Autodesk Fusion 360 part; units mm, degrees
(part 2 of 5)
  spline S371 degree 3 poles (-22.5351, -2.4516) (-22.49, -2.4245) (-22.4449, -2.4426) (-22.4449, -2.4877) knots 0 0 0 0 1 1 1 1
  spline S372 degree 3 poles (-22.4449, -2.4877) (-22.4449, -2.5419) (-22.49, -2.587) (-22.5351, -2.587) knots 0 0 0 0 1 1 1 1
  spline S373 degree 3 poles (-22.5351, -2.587) (-22.5893, -2.587) (-22.6254, -2.5689) (-22.6254, -2.5509) knots 0 0 0 0 1 1 1 1
  spline S374 degree 3 poles (-18.0948, -1.7747) (-17.9685, -1.7386) (-17.806, -1.6755) (-17.7338, -1.6303) knots 0 0 0 0 1 1 1 1
  spline S375 degree 3 poles (-17.7338, -1.6303) (-17.6436, -1.5762) (-17.6436, -1.5942) (-17.7429, -1.7116) knots 0 0 0 0 1 1 1 1
  spline S376 degree 3 poles (-17.7429, -1.7116) (-17.806, -1.7928) (-17.9685, -1.865) (-18.1039, -1.856) knots 0 0 0 0 1 1 1 1
  line L50 (-18.1039, -1.856) -> (-18.3385, -1.8469)
  line L51 (-18.3385, -1.8469) -> (-18.0948, -1.7747)
  spline S377 degree 3 poles (-20.1345, -1.7838) (-20.1616, -1.7386) (-20.0533, -1.6845) (-19.8908, -1.6574) knots 0 0 0 0 1 1 1 1
  spline S378 degree 3 poles (-19.8908, -1.6574) (-19.5569, -1.6123) (-19.4576, -1.6574) (-19.6471, -1.7747) knots 0 0 0 0 1 1 1 1
  spline S379 degree 3 poles (-19.6471, -1.7747) (-19.8186, -1.883) (-20.0713, -1.8921) (-20.1345, -1.7838) knots 0 0 0 0 1 1 1 1
  spline S380 degree 3 poles (-21.9034, -1.6845) (-22.0027, -1.6213) (-21.9666, -1.5942) (-21.7409, -1.5942) knots 0 0 0 0 1 1 1 1
  spline S381 degree 3 poles (-21.7409, -1.5942) (-21.5604, -1.5942) (-21.4612, -1.6303) (-21.4973, -1.6845) knots 0 0 0 0 1 1 1 1
  spline S382 degree 3 poles (-21.4973, -1.6845) (-21.5695, -1.8018) (-21.7319, -1.8018) (-21.9034, -1.6845) knots 0 0 0 0 1 1 1 1
  spline S383 degree 3 poles (-27.887, -1.5401) (-28.7714, -1.3957) (-29.1595, -1.2332) (-29.3129, -0.9444) knots 0 0 0 0 1 1 1 1
  spline S384 degree 3 poles (-29.3129, -0.9444) (-29.4032, -0.782) (-29.3851, -0.7278) (-29.2497, -0.6286) knots 0 0 0 0 1 1 1 1
  spline S385 degree 3 poles (-29.2497, -0.6286) (-29.1053, -0.5203) (-29.0692, -0.5383) (-28.97, -0.7369) knots 0 0 0 0 1 1 1 1
  spline S386 degree 3 poles (-28.97, -0.7369) (-28.8887, -0.8813) (-28.7714, -0.9625) (-28.636, -0.9625) knots 0 0 0 0 1 1 1 1
  spline S387 degree 3 poles (-28.636, -0.9625) (-28.5187, -0.9625) (-28.3021, -1.0257) (-28.1667, -1.0979) knots 0 0 0 0 1 1 1 1
  spline S388 degree 3 poles (-28.1667, -1.0979) (-27.8689, -1.2513) (-26.9935, -1.2784) (-26.9123, -1.143) knots 0 0 0 0 1 1 1 1
  spline S389 degree 3 poles (-26.9123, -1.143) (-26.8762, -1.0888) (-27.0386, -1.0527) (-27.3455, -1.0527) knots 0 0 0 0 1 1 1 1
  spline S390 degree 3 poles (-27.3455, -1.0527) (-27.7065, -1.0527) (-27.8689, -1.0076) (-27.9862, -0.8813) knots 0 0 0 0 1 1 1 1
  spline S391 degree 3 poles (-27.9862, -0.8813) (-28.0765, -0.791) (-28.2841, -0.6827) (-28.4555, -0.6556) knots 0 0 0 0 1 1 1 1
  spline S392 degree 3 poles (-28.4555, -0.6556) (-28.8346, -0.5834) (-28.8436, -0.4481) (-28.4916, -0.06) knots 0 0 0 0 1 1 1 1
  spline S393 degree 3 poles (-28.4916, -0.06) (-28.3382, 0.1115) (-28.1938, 0.3461) (-28.1577, 0.4635) knots 0 0 0 0 1 1 1 1
  spline S394 degree 3 poles (-28.1577, 0.4635) (-28.1126, 0.644) (-28.0675, 0.662) (-27.8689, 0.6079) knots 0 0 0 0 1 1 1 1
  spline S395 degree 3 poles (-27.8689, 0.6079) (-27.7426, 0.5718) (-27.526, 0.5537) (-27.3816, 0.5627) knots 0 0 0 0 1 1 1 1
  spline S396 degree 3 poles (-27.3816, 0.5627) (-27.0928, 0.5808) (-26.7137, 0.3552) (-26.6686, 0.1386) knots 0 0 0 0 1 1 1 1
  spline S397 degree 3 poles (-26.6686, 0.1386) (-26.6325, -0.069) (-25.748, -0.0961) (-24.8907, 0.0934) knots 0 0 0 0 1 1 1 1
  spline S398 degree 3 poles (-24.8907, 0.0934) (-24.2679, 0.2288) (-24.2048, 0.2288) (-23.9611, 0.0754) knots 0 0 0 0 1 1 1 1
  spline S399 degree 3 poles (-23.9611, 0.0754) (-23.7535, -0.0419) (-23.6633, -0.051) (-23.5911, 0.0303) knots 0 0 0 0 1 1 1 1
  spline S400 degree 3 poles (-23.5911, 0.0303) (-23.5098, 0.1115) (-23.5189, 0.1566) (-23.6452, 0.2469) knots 0 0 0 0 1 1 1 1
  spline S401 degree 3 poles (-23.6452, 0.2469) (-23.8347, 0.3913) (-23.8347, 0.4454) (-23.6633, 0.5176) knots 0 0 0 0 1 1 1 1
  spline S402 degree 3 poles (-23.6633, 0.5176) (-23.5279, 0.5627) (-23.0766, 0.1927) (-23.0766, 0.0303) knots 0 0 0 0 1 1 1 1
  spline S403 degree 3 poles (-23.0766, 0.0303) (-23.0766, -0.078) (-22.9774, -0.078) (-22.8149, 0.0212) knots 0 0 0 0 1 1 1 1
  spline S404 degree 3 poles (-22.8149, 0.0212) (-22.7517, 0.0664) (-22.7247, 0.1476) (-22.7517, 0.2017) knots 0 0 0 0 1 1 1 1
  spline S405 degree 3 poles (-22.7517, 0.2017) (-22.7878, 0.2559) (-22.7247, 0.3371) (-22.5893, 0.3913) knots 0 0 0 0 1 1 1 1
  spline S406 degree 3 poles (-22.5893, 0.3913) (-22.3185, 0.4905) (-22.2915, 0.7071) (-22.499, 0.9418) knots 0 0 0 0 1 1 1 1
  spline S407 degree 3 poles (-22.499, 0.9418) (-22.6344, 1.0862) (-22.6254, 1.1313) (-22.3456, 1.4652) knots 0 0 0 0 1 1 1 1
  spline S408 degree 3 poles (-22.3456, 1.4652) (-22.1832, 1.6728) (-21.9846, 1.8353) (-21.9034, 1.8353) knots 0 0 0 0 1 1 1 1
  spline S409 degree 3 poles (-21.9034, 1.8353) (-21.6687, 1.8353) (-21.4973, 2.0789) (-21.6236, 2.2324) knots 0 0 0 0 1 1 1 1
  spline S410 degree 3 poles (-21.6236, 2.2324) (-21.8131, 2.458) (-21.4251, 3.8027) (-21.1543, 3.8388) knots 0 0 0 0 1 1 1 1
  spline S411 degree 3 poles (-21.1543, 3.8388) (-21.1002, 3.8388) (-19.9901, 3.8569) (-18.6995, 3.8659) knots 0 0 0 0 1 1 1 1
  spline S412 degree 3 poles (-18.6995, 3.8659) (-17.4089, 3.8749) (-15.8566, 3.92) (-15.261, 3.9561) knots 0 0 0 0 1 1 1 1
  spline S413 degree 3 poles (-15.261, 3.9561) (-14.6563, 3.9922) (-14.0877, 4.0013) (-14.0065, 3.9652) knots 0 0 0 0 1 1 1 1
  spline S414 degree 3 poles (-14.0065, 3.9652) (-13.8531, 3.911) (-13.8531, 3.902) (-13.9975, 3.7395) knots 0 0 0 0 1 1 1 1
  spline S415 degree 3 poles (-13.9975, 3.7395) (-14.187, 3.532) (-14.3134, 3.4959) (-15.5678, 3.3334) knots 0 0 0 0 1 1 1 1
  spline S416 degree 3 poles (-15.5678, 3.3334) (-16.5967, 3.198) (-17.1111, 3.0085) (-17.436, 2.6475) knots 0 0 0 0 1 1 1 1
  spline S417 degree 3 poles (-17.436, 2.6475) (-17.7158, 2.3316) (-19.3222, 1.5645) (-19.6923, 1.5645) knots 0 0 0 0 1 1 1 1
  spline S418 degree 3 poles (-19.6923, 1.5645) (-20.0172, 1.5645) (-20.5496, 1.3479) (-20.5496, 1.2216) knots 0 0 0 0 1 1 1 1
  spline S419 degree 3 poles (-20.5496, 1.2216) (-20.5496, 1.1855) (-20.6399, 1.1133) (-20.7572, 1.0681) knots 0 0 0 0 1 1 1 1
  spline S420 degree 3 poles (-20.7572, 1.0681) (-20.8655, 1.014) (-21.0641, 0.7613) (-21.1994, 0.4905) knots 0 0 0 0 1 1 1 1
  spline S421 degree 3 poles (-21.1994, 0.4905) (-21.5334, -0.1683) (-21.8131, -0.439) (-22.5351, -0.8181) knots 0 0 0 0 1 1 1 1
  spline S422 degree 3 poles (-22.5351, -0.8181) (-23.1398, -1.143) (-24.4665, -1.6394) (-24.8816, -1.7025) knots 0 0 0 0 1 1 1 1
  spline S423 degree 3 poles (-24.8816, -1.7025) (-25.2878, -1.7747) (-27.0747, -1.6755) (-27.887, -1.5401) knots 0 0 0 0 1 1 1 1
  spline S424 degree 3 poles (-18.0226, -1.4589) (-17.9595, -1.3867) (-17.8692, -1.3235) (-17.8241, -1.3235) knots 0 0 0 0 1 1 1 1
  spline S425 degree 3 poles (-17.8241, -1.3235) (-17.7699, -1.3235) (-17.779, -1.3867) (-17.8421, -1.4589) knots 0 0 0 0 1 1 1 1
  spline S426 degree 3 poles (-17.8421, -1.4589) (-17.9053, -1.5311) (-17.9956, -1.5942) (-18.0407, -1.5942) knots 0 0 0 0 1 1 1 1
  spline S427 degree 3 poles (-18.0407, -1.5942) (-18.0948, -1.5942) (-18.0858, -1.5311) (-18.0226, -1.4589) knots 0 0 0 0 1 1 1 1
  spline S428 degree 3 poles (-20.0081, -1.5581) (-20.0081, -1.5401) (-19.945, -1.495) (-19.8637, -1.4679) knots 0 0 0 0 1 1 1 1
  spline S429 degree 3 poles (-19.8637, -1.4679) (-19.7915, -1.4408) (-19.7554, -1.4498) (-19.7825, -1.504) knots 0 0 0 0 1 1 1 1
  spline S430 degree 3 poles (-19.7825, -1.504) (-19.8367, -1.5942) (-20.0081, -1.6303) (-20.0081, -1.5581) knots 0 0 0 0 1 1 1 1
  spline S431 degree 3 poles (-18.3836, -1.3506) (-18.3114, -1.3235) (-18.167, -1.2603) (-18.0678, -1.2062) knots 0 0 0 0 1 1 1 1
  spline S432 degree 3 poles (-18.0678, -1.2062) (-17.9053, -1.1249) (-17.8963, -1.1249) (-18.0136, -1.2603) knots 0 0 0 0 1 1 1 1
  spline S433 degree 3 poles (-18.0136, -1.2603) (-18.0768, -1.3506) (-18.2212, -1.4137) (-18.3295, -1.4047) knots 0 0 0 0 1 1 1 1
  spline S434 degree 3 poles (-18.3295, -1.4047) (-18.4558, -1.4047) (-18.4739, -1.3867) (-18.3836, -1.3506) knots 0 0 0 0 1 1 1 1
  spline S435 degree 3 poles (-20.324, -1.3325) (-20.2699, -1.2964) (-20.1164, -1.2332) (-19.963, -1.1971) knots 0 0 0 0 1 1 1 1
  spline S436 degree 3 poles (-19.963, -1.1971) (-19.7103, -1.143) (-19.7013, -1.152) (-19.8637, -1.2784) knots 0 0 0 0 1 1 1 1
  spline S437 degree 3 poles (-19.8637, -1.2784) (-20.0533, -1.4228) (-20.4684, -1.4769) (-20.324, -1.3325) knots 0 0 0 0 1 1 1 1
  spline S438 degree 3 poles (-21.8402, -1.3506) (-21.777, -1.3325) (-21.6687, -1.3325) (-21.6146, -1.3506) knots 0 0 0 0 1 1 1 1
  spline S439 degree 3 poles (-21.6146, -1.3506) (-21.5514, -1.3776) (-21.5965, -1.3957) (-21.7229, -1.3957) knots 0 0 0 0 1 1 1 1
  spline S440 degree 3 poles (-21.7229, -1.3957) (-21.8492, -1.3957) (-21.8944, -1.3776) (-21.8402, -1.3506) knots 0 0 0 0 1 1 1 1
  spline S441 degree 3 poles (17.4817, -1.0979) (16.2363, -0.8452) (15.8662, -0.6286) (15.3518, 0.1205) knots 0 0 0 0 1 1 1 1
  spline S442 degree 3 poles (15.3518, 0.1205) (14.9096, 0.7703) (14.5125, 1.6096) (14.4313, 2.0609) knots 0 0 0 0 1 1 1 1
  spline S443 degree 3 poles (14.4313, 2.0609) (14.3952, 2.2594) (14.2688, 2.5663) (14.1515, 2.7378) knots 0 0 0 0 1 1 1 1
  spline S444 degree 3 poles (14.1515, 2.7378) (13.9981, 2.9724) (13.9259, 3.2432) (13.8807, 3.7486) knots 0 0 0 0 1 1 1 1
  line L52 (13.8807, 3.7486) -> (13.8176, 4.4525)
  line L53 (13.8176, 4.4525) -> (14.0973, 4.4525)
  spline S445 degree 3 poles (14.0973, 4.4525) (14.6749, 4.4525) (14.7381, 4.3532) (14.7381, 3.4778) knots 0 0 0 0 1 1 1 1
  spline S446 degree 3 poles (14.7381, 3.4778) (14.7381, 3.0266) (14.693, 2.6385) (14.6388, 2.5843) knots 0 0 0 0 1 1 1 1
  spline S447 degree 3 poles (14.6388, 2.5843) (14.5305, 2.476) (14.8013, 1.8533) (15.0991, 1.5194) knots 0 0 0 0 1 1 1 1
  spline S448 degree 3 poles (15.0991, 1.5194) (15.1803, 1.4201) (15.3338, 1.2216) (15.424, 1.0681) knots 0 0 0 0 1 1 1 1
  spline S449 degree 3 poles (15.424, 1.0681) (15.5774, 0.8245) (15.5865, 0.8064) (15.433, 0.8696) knots 0 0 0 0 1 1 1 1
  spline S450 degree 3 poles (15.433, 0.8696) (15.3247, 0.9057) (15.2796, 0.8876) (15.2796, 0.7884) knots 0 0 0 0 1 1 1 1
  spline S451 degree 3 poles (15.2796, 0.7884) (15.2796, 0.6801) (15.3338, 0.653) (15.4872, 0.6891) knots 0 0 0 0 1 1 1 1
  spline S452 degree 3 poles (15.4872, 0.6891) (15.5955, 0.7252) (15.7489, 0.7071) (15.8211, 0.662) knots 0 0 0 0 1 1 1 1
  spline S453 degree 3 poles (15.8211, 0.662) (15.9114, 0.5988) (15.9204, 0.5718) (15.8392, 0.5718) knots 0 0 0 0 1 1 1 1
  spline S454 degree 3 poles (15.8392, 0.5718) (15.6587, 0.5718) (15.7218, 0.4454) (15.9655, 0.3281) knots 0 0 0 0 1 1 1 1
  spline S455 degree 3 poles (15.9655, 0.3281) (16.0919, 0.2739) (16.2543, 0.2469) (16.3265, 0.2739) knots 0 0 0 0 1 1 1 1
  spline S456 degree 3 poles (16.3265, 0.2739) (16.3987, 0.301) (16.507, 0.283) (16.5702, 0.2288) knots 0 0 0 0 1 1 1 1
  spline S457 degree 3 poles (16.5702, 0.2288) (16.6243, 0.1837) (17.0034, 0.0122) (17.4005, -0.1502) knots 0 0 0 0 1 1 1 1
  spline S458 degree 3 poles (17.4005, -0.1502) (18.0593, -0.412) (18.1947, -0.43) (19.0701, -0.421) knots 0 0 0 0 1 1 1 1
  spline S459 degree 3 poles (19.0701, -0.421) (19.5936, -0.412) (20.126, -0.412) (20.2614, -0.421) knots 0 0 0 0 1 1 1 1
  spline S460 degree 3 poles (20.2614, -0.421) (20.6765, -0.439) (21.1097, -0.3939) (20.9744, -0.3488) knots 0 0 0 0 1 1 1 1
  spline S461 degree 3 poles (20.9744, -0.3488) (20.8841, -0.3217) (20.9022, -0.2585) (21.0646, -0.1322) knots 0 0 0 0 1 1 1 1
  spline S462 degree 3 poles (21.0646, -0.1322) (21.218, -0.0058) (21.2361, 0.0303) (21.1188, -0.0058) knots 0 0 0 0 1 1 1 1
  spline S463 degree 3 poles (21.1188, -0.0058) (20.83, -0.0961) (20.848, 0.1927) (21.1458, 0.5627) knots 0 0 0 0 1 1 1 1
  spline S464 degree 3 poles (21.1458, 0.5627) (21.3805, 0.8425) (21.5068, 0.9328) (21.7686, 0.9508) knots 0 0 0 0 1 1 1 1
  spline S465 degree 3 poles (21.7686, 0.9508) (22.0574, 0.9779) (22.0935, 1.005) (22.0754, 1.2216) knots 0 0 0 0 1 1 1 1
  spline S466 degree 3 poles (22.0754, 1.2216) (22.0664, 1.393) (22.1115, 1.4743) (22.2559, 1.5194) knots 0 0 0 0 1 1 1 1
  spline S467 degree 3 poles (22.2559, 1.5194) (22.4274, 1.5735) (22.4364, 1.5916) (22.292, 1.6277) knots 0 0 0 0 1 1 1 1
  spline S468 degree 3 poles (22.292, 1.6277) (22.1025, 1.6728) (22.0844, 1.9797) (22.274, 2.0519) knots 0 0 0 0 1 1 1 1
  spline S469 degree 3 poles (22.274, 2.0519) (22.3462, 2.0789) (22.4003, 2.1872) (22.3823, 2.3046) knots 0 0 0 0 1 1 1 1
  spline S470 degree 3 poles (22.3823, 2.3046) (22.3642, 2.476) (22.4093, 2.5121) (22.6259, 2.5121) knots 0 0 0 0 1 1 1 1
  spline S471 degree 3 poles (22.6259, 2.5121) (22.7794, 2.5212) (23.023, 2.6385) (23.2306, 2.819) knots 0 0 0 0 1 1 1 1
  spline S472 degree 3 poles (23.2306, 2.819) (23.5375, 3.0717) (23.6458, 3.1078) (24.0158, 3.0897) knots 0 0 0 0 1 1 1 1
  spline S473 degree 3 poles (24.0158, 3.0897) (24.2504, 3.0807) (24.5483, 3.1258) (24.6746, 3.189) knots 0 0 0 0 1 1 1 1
  spline S474 degree 3 poles (24.6746, 3.189) (24.8732, 3.2793) (24.9634, 3.2702) (25.2071, 3.1439) knots 0 0 0 0 1 1 1 1
  spline S475 degree 3 poles (25.2071, 3.1439) (25.3786, 3.0536) (25.5861, 3.0175) (25.7215, 3.0536) knots 0 0 0 0 1 1 1 1
  spline S476 degree 3 poles (25.7215, 3.0536) (26.1276, 3.1529) (25.902, 2.8822) (25.4237, 2.7017) knots 0 0 0 0 1 1 1 1
  spline S477 degree 3 poles (25.4237, 2.7017) (24.4129, 2.3136) (24.2775, 2.2324) (23.8804, 1.7721) knots 0 0 0 0 1 1 1 1
  spline S478 degree 3 poles (23.8804, 1.7721) (23.6367, 1.4923) (23.3028, 1.2216) (23.0772, 1.1223) knots 0 0 0 0 1 1 1 1
  spline S479 degree 3 poles (23.0772, 1.1223) (22.8425, 1.014) (22.635, 0.8425) (22.5537, 0.6801) knots 0 0 0 0 1 1 1 1
  spline S480 degree 3 poles (22.5537, 0.6801) (22.3913, 0.3642) (21.3263, -0.5654) (20.9744, -0.7098) knots 0 0 0 0 1 1 1 1
  spline S481 degree 3 poles (20.9744, -0.7098) (20.0358, -1.0798) (19.2416, -1.3235) (18.9257, -1.3235) knots 0 0 0 0 1 1 1 1
  spline S482 degree 3 poles (18.9257, -1.3235) (18.7181, -1.3235) (18.0683, -1.2242) (17.4817, -1.0979) knots 0 0 0 0 1 1 1 1
  spline S483 degree 3 poles (-18.3836, -1.0979) (-18.0858, -0.9264) (-17.9324, -0.9354) (-18.149, -1.0979) knots 0 0 0 0 1 1 1 1
  spline S484 degree 3 poles (-18.149, -1.0979) (-18.2483, -1.1701) (-18.3927, -1.2332) (-18.4649, -1.2332) knots 0 0 0 0 1 1 1 1
  spline S485 degree 3 poles (-18.4649, -1.2332) (-18.5551, -1.2242) (-18.528, -1.1791) (-18.3836, -1.0979) knots 0 0 0 0 1 1 1 1
  spline S486 degree 3 poles (-22.0839, -1.143) (-22.0839, -1.0979) (-21.9756, -1.0527) (-21.8402, -1.0527) knots 0 0 0 0 1 1 1 1
  spline S487 degree 3 poles (-21.8402, -1.0527) (-21.6417, -1.0527) (-21.6146, -1.0708) (-21.7229, -1.143) knots 0 0 0 0 1 1 1 1
  spline S488 degree 3 poles (-21.7229, -1.143) (-21.9034, -1.2603) (-22.0839, -1.2603) (-22.0839, -1.143) knots 0 0 0 0 1 1 1 1
  spline S489 degree 3 poles (-20.2338, -1.0076) (-20.0894, -0.9444) (-19.945, -0.9083) (-19.9179, -0.9264) knots 0 0 0 0 1 1 1 1
  spline S490 degree 3 poles (-19.9179, -0.9264) (-19.8547, -0.9986) (-20.1345, -1.143) (-20.324, -1.134) knots 0 0 0 0 1 1 1 1
  spline S491 degree 3 poles (-20.324, -1.134) (-20.4594, -1.134) (-20.4413, -1.0979) (-20.2338, -1.0076) knots 0 0 0 0 1 1 1 1
  spline S492 degree 3 poles (-21.4341, -0.8813) (-21.5063, -0.6827) (-21.4973, -0.5744) (-21.398, -0.43) knots 0 0 0 0 1 1 1 1
  spline S493 degree 3 poles (-21.398, -0.43) (-21.1994, -0.1593) (-21.1272, -0.1954) (-21.0189, -0.6195) knots 0 0 0 0 1 1 1 1
  spline S494 degree 3 poles (-21.0189, -0.6195) (-20.9467, -0.9083) (-20.9467, -1.0166) (-21.028, -1.0708) knots 0 0 0 0 1 1 1 1
  spline S495 degree 3 poles (-21.028, -1.0708) (-21.2265, -1.1971) (-21.3438, -1.143) (-21.4341, -0.8813) knots 0 0 0 0 1 1 1 1
  spline S496 degree 3 poles (-18.6544, -0.9896) (-18.5822, -0.9625) (-18.4107, -0.8813) (-18.2753, -0.8091) knots 0 0 0 0 1 1 1 1
  spline S497 degree 3 poles (-18.2753, -0.8091) (-18.1309, -0.7459) (-18.0226, -0.7098) (-18.0226, -0.7278) knots 0 0 0 0 1 1 1 1
  spline S498 degree 3 poles (-18.0226, -0.7278) (-18.0226, -0.8091) (-18.51, -1.0437) (-18.6544, -1.0437) knots 0 0 0 0 1 1 1 1
  spline S499 degree 3 poles (-18.6544, -1.0437) (-18.7717, -1.0347) (-18.7717, -1.0347) (-18.6544, -0.9896) knots 0 0 0 0 1 1 1 1
  spline S500 degree 3 poles (-20.3691, -0.7459) (-20.0352, -0.6195) (-19.8818, -0.6466) (-20.0984, -0.782) knots 0 0 0 0 1 1 1 1
  spline S501 degree 3 poles (-20.0984, -0.782) (-20.1706, -0.8361) (-20.333, -0.8632) (-20.4594, -0.8632) knots 0 0 0 0 1 1 1 1
  spline S502 degree 3 poles (-20.4594, -0.8632) (-20.6579, -0.8632) (-20.6489, -0.8452) (-20.3691, -0.7459) knots 0 0 0 0 1 1 1 1
  spline S503 degree 3 poles (-18.4739, -0.7098) (-18.4739, -0.5925) (-18.3656, -0.5112) (-18.2753, -0.5654) knots 0 0 0 0 1 1 1 1
  spline S504 degree 3 poles (-18.2753, -0.5654) (-18.1851, -0.6195) (-18.2663, -0.782) (-18.3927, -0.782) knots 0 0 0 0 1 1 1 1
  spline S505 degree 3 poles (-18.3927, -0.782) (-18.4378, -0.782) (-18.4739, -0.7459) (-18.4739, -0.7098) knots 0 0 0 0 1 1 1 1
  spline S506 degree 3 poles (-20.4143, -0.5112) (-20.3872, -0.4661) (-20.2879, -0.421) (-20.2067, -0.421) knots 0 0 0 0 1 1 1 1
  spline S507 degree 3 poles (-20.2067, -0.421) (-20.0713, -0.421) (-20.0713, -0.439) (-20.1886, -0.5112) knots 0 0 0 0 1 1 1 1
  spline S508 degree 3 poles (-20.1886, -0.5112) (-20.3691, -0.6286) (-20.4865, -0.6286) (-20.4143, -0.5112) knots 0 0 0 0 1 1 1 1
  spline S509 degree 3 poles (-30.3869, -0.3307) (-30.8111, -0.1141) (-31.0277, 0.2649) (-31.0547, 0.8245) knots 0 0 0 0 1 1 1 1
  spline S510 degree 3 poles (-31.0547, 0.8245) (-31.0638, 1.1674) (-31.0277, 1.2486) (-30.8111, 1.4111) knots 0 0 0 0 1 1 1 1
  line L54 (-30.8111, 1.4111) -> (-30.5674, 1.6006)
  line L55 (-30.5674, 1.6006) -> (-30.3598, 1.393)
  spline S511 degree 3 poles (-30.3598, 1.393) (-30.2244, 1.2486) (-30.1974, 1.1674) (-30.2696, 1.1403) knots 0 0 0 0 1 1 1 1
  spline S512 degree 3 poles (-30.2696, 1.1403) (-30.3327, 1.1223) (-30.4771, 1.023) (-30.5854, 0.9328) knots 0 0 0 0 1 1 1 1
  line L56 (-30.5854, 0.9328) -> (-30.793, 0.7613)
  line L57 (-30.793, 0.7613) -> (-30.5945, 0.7523)
  spline S513 degree 3 poles (-30.5945, 0.7523) (-30.3508, 0.7523) (-30.3237, 0.644) (-30.5223, 0.4815) knots 0 0 0 0 1 1 1 1
  spline S514 degree 3 poles (-30.5223, 0.4815) (-30.7298, 0.31) (-30.6847, 0.2108) (-30.3779, 0.2108) knots 0 0 0 0 1 1 1 1
  spline S515 degree 3 poles (-30.3779, 0.2108) (-30.1432, 0.2108) (-30.1161, 0.1837) (-30.1613, 0.0212) knots 0 0 0 0 1 1 1 1
  spline S516 degree 3 poles (-30.1613, 0.0212) (-30.2154, -0.1502) (-30.1974, -0.1593) (-29.9447, -0.1051) knots 0 0 0 0 1 1 1 1
  spline S517 degree 3 poles (-29.9447, -0.1051) (-29.692, -0.051) (-29.6649, -0.069) (-29.6649, -0.2766) knots 0 0 0 0 1 1 1 1
  spline S518 degree 3 poles (-29.6649, -0.2766) (-29.6649, -0.5744) (-29.8905, -0.5834) (-30.3869, -0.3307) knots 0 0 0 0 1 1 1 1
  spline S519 degree 3 poles (-29.8273, 1.0952) (-30.2876, 1.6548) (-30.3057, 1.8082) (-29.8995, 1.8894) knots 0 0 0 0 1 1 1 1
  spline S520 degree 3 poles (-29.8995, 1.8894) (-29.4663, 1.9616) (-29.1144, 1.8714) (-28.7624, 1.5735) knots 0 0 0 0 1 1 1 1
  spline S521 degree 3 poles (-28.7624, 1.5735) (-28.4916, 1.3479) (-28.4646, 1.2847) (-28.4826, 0.8606) knots 0 0 0 0 1 1 1 1
  spline S522 degree 3 poles (-28.4826, 0.8606) (-28.5007, 0.2017) (-28.618, -0.0239) (-29.0061, -0.2315) knots 0 0 0 0 1 1 1 1
  line L58 (-29.0061, -0.2315) -> (-29.349, -0.4029)
  line L59 (-29.349, -0.4029) -> (-29.3941, 0.1205)
  spline S523 degree 3 poles (-29.3941, 0.1205) (-29.4302, 0.5718) (-29.4934, 0.7071) (-29.8273, 1.0952) knots 0 0 0 0 1 1 1 1
  spline S524 degree 3 poles (-20.8204, -0.2495) (-20.8204, -0.1773) (-20.2699, -0.051) (-20.1977, -0.1141) knots 0 0 0 0 1 1 1 1
  spline S525 degree 3 poles (-20.1977, -0.1141) (-20.1886, -0.1232) (-20.1977, -0.1773) (-20.2338, -0.2315) knots 0 0 0 0 1 1 1 1
  spline S526 degree 3 poles (-20.2338, -0.2315) (-20.306, -0.3488) (-20.8204, -0.3668) (-20.8204, -0.2495) knots 0 0 0 0 1 1 1 1
  spline S527 degree 3 poles (-14.7736, 0.0303) (-14.6924, 0.1837) (-14.6473, 0.1927) (-14.5029, 0.1025) knots 0 0 0 0 1 1 1 1
  spline S528 degree 3 poles (-14.5029, 0.1025) (-14.2863, -0.0329) (-14.3585, -0.1502) (-14.6473, -0.1502) knots 0 0 0 0 1 1 1 1
  spline S529 degree 3 poles (-14.6473, -0.1502) (-14.8458, -0.1502) (-14.8549, -0.1232) (-14.7736, 0.0303) knots 0 0 0 0 1 1 1 1
  spline S530 degree 3 poles (-15.6761, 0.0393) (-16.0823, 0.2649) (-16.4884, 0.8696) (-16.4884, 1.2486) knots 0 0 0 0 1 1 1 1
  spline S531 degree 3 poles (-16.4884, 1.2486) (-16.4884, 1.6728) (-16.3079, 2.2233) (-16.1003, 2.4399) knots 0 0 0 0 1 1 1 1
  spline S532 degree 3 poles (-16.1003, 2.4399) (-15.8657, 2.7017) (-15.8386, 2.7017) (-15.6581, 2.3858) knots 0 0 0 0 1 1 1 1
  line L60 (-15.6581, 2.3858) -> (-15.5137, 2.1241)
  line L61 (-15.5137, 2.1241) -> (-15.7935, 2.1602)
  spline S533 degree 3 poles (-15.7935, 2.1602) (-16.0371, 2.2053) (-16.1003, 2.1692) (-16.1906, 1.9616) knots 0 0 0 0 1 1 1 1
  spline S534 degree 3 poles (-16.1906, 1.9616) (-16.2718, 1.7811) (-16.2808, 1.6818) (-16.2086, 1.5916) knots 0 0 0 0 1 1 1 1
  spline S535 degree 3 poles (-16.2086, 1.5916) (-16.1364, 1.5104) (-16.1364, 1.4743) (-16.2086, 1.4743) knots 0 0 0 0 1 1 1 1
  spline S536 degree 3 poles (-16.2086, 1.4743) (-16.2628, 1.4743) (-16.3079, 1.393) (-16.3079, 1.2938) knots 0 0 0 0 1 1 1 1
  spline S537 degree 3 poles (-16.3079, 1.2938) (-16.3079, 1.1674) (-16.2447, 1.1133) (-16.1093, 1.1133) knots 0 0 0 0 1 1 1 1
  spline S538 degree 3 poles (-16.1093, 1.1133) (-15.9288, 1.1133) (-15.9288, 1.1042) (-16.0732, 0.9418) knots 0 0 0 0 1 1 1 1
  spline S539 degree 3 poles (-16.0732, 0.9418) (-16.2447, 0.7523) (-16.1996, 0.5718) (-15.983, 0.5718) knots 0 0 0 0 1 1 1 1
  spline S540 degree 3 poles (-15.983, 0.5718) (-15.9108, 0.5718) (-15.8566, 0.4905) (-15.8566, 0.3913) knots 0 0 0 0 1 1 1 1
  spline S541 degree 3 poles (-15.8566, 0.3913) (-15.8566, 0.2739) (-15.7935, 0.2108) (-15.6852, 0.2108) knots 0 0 0 0 1 1 1 1
  spline S542 degree 3 poles (-15.6852, 0.2108) (-15.5859, 0.2108) (-15.4956, 0.1566) (-15.4686, 0.0934) knots 0 0 0 0 1 1 1 1
  spline S543 degree 3 poles (-15.4686, 0.0934) (-15.4325, 0.0032) (-15.4054, 0.0032) (-15.3061, 0.0934) knots 0 0 0 0 1 1 1 1
  spline S544 degree 3 poles (-15.3061, 0.0934) (-15.1437, 0.2559) (-15.0715, 0.2378) (-15.0173, 0.0303) knots 0 0 0 0 1 1 1 1
  spline S545 degree 3 poles (-15.0173, 0.0303) (-14.9541, -0.2134) (-15.2339, -0.2134) (-15.6761, 0.0393) knots 0 0 0 0 1 1 1 1
  spline S546 degree 3 poles (-20.8204, 0.0212) (-20.8204, 0.0664) (-20.7211, 0.1205) (-20.5948, 0.1386) knots 0 0 0 0 1 1 1 1
  spline S547 degree 3 poles (-20.5948, 0.1386) (-20.3601, 0.1837) (-20.2789, 0.0844) (-20.4865, 0.0032) knots 0 0 0 0 1 1 1 1
  spline S548 degree 3 poles (-20.4865, 0.0032) (-20.667, -0.078) (-20.8204, -0.069) (-20.8204, 0.0212) knots 0 0 0 0 1 1 1 1
  spline S549 degree 3 poles (-14.2321, 0.3732) (-14.2321, 0.4544) (-14.169, 0.4454) (-13.9975, 0.3281) knots 0 0 0 0 1 1 1 1
  spline S550 degree 3 poles (-13.9975, 0.3281) (-13.7809, 0.1927) (-13.7719, 0.1747) (-13.9253, 0.1115) knots 0 0 0 0 1 1 1 1
  spline S551 degree 3 poles (-13.9253, 0.1115) (-14.0968, 0.0573) (-14.2321, 0.1656) (-14.2321, 0.3732) knots 0 0 0 0 1 1 1 1
  spline S552 degree 3 poles (-19.232, 0.31) (-19.2049, 0.3552) (-19.1417, 0.3732) (-19.0966, 0.3371) knots 0 0 0 0 1 1 1 1
  spline S553 degree 3 poles (-19.0966, 0.3371) (-19.0515, 0.31) (-19.0334, 0.2469) (-19.0695, 0.2017) knots 0 0 0 0 1 1 1 1
  spline S554 degree 3 poles (-19.0695, 0.2017) (-19.0966, 0.1566) (-19.1598, 0.1386) (-19.2049, 0.1747) knots 0 0 0 0 1 1 1 1
  spline S555 degree 3 poles (-19.2049, 0.1747) (-19.25, 0.2017) (-19.2681, 0.2649) (-19.232, 0.31) knots 0 0 0 0 1 1 1 1
  spline S556 degree 3 poles (-14.5029, 0.3913) (-14.557, 0.4905) (-14.5751, 0.5718) (-14.557, 0.5718) knots 0 0 0 0 1 1 1 1
  spline S557 degree 3 poles (-14.557, 0.5718) (-14.53, 0.5718) (-14.4668, 0.4905) (-14.4126, 0.3913) knots 0 0 0 0 1 1 1 1
  spline S558 degree 3 poles (-14.4126, 0.3913) (-14.3585, 0.292) (-14.3404, 0.2108) (-14.3585, 0.2108) knots 0 0 0 0 1 1 1 1
  spline S559 degree 3 poles (-14.3585, 0.2108) (-14.3856, 0.2108) (-14.4487, 0.292) (-14.5029, 0.3913) knots 0 0 0 0 1 1 1 1
  spline S560 degree 3 poles (-20.8655, 0.292) (-20.7211, 0.4183) (-20.3691, 0.4996) (-20.3691, 0.4003) knots 0 0 0 0 1 1 1 1
  spline S561 degree 3 poles (-20.3691, 0.4003) (-20.3691, 0.3191) (-20.5496, 0.2469) (-20.8204, 0.2198) knots 0 0 0 0 1 1 1 1
  spline S562 degree 3 poles (-20.8204, 0.2198) (-20.8926, 0.2108) (-20.9106, 0.2378) (-20.8655, 0.292) knots 0 0 0 0 1 1 1 1
  spline S563 degree 3 poles (-14.9271, 0.5898) (-14.9, 0.653) (-14.8819, 0.6079) (-14.8819, 0.4815) knots 0 0 0 0 1 1 1 1
  spline S564 degree 3 poles (-14.8819, 0.4815) (-14.8819, 0.3552) (-14.9, 0.31) (-14.9271, 0.3642) knots 0 0 0 0 1 1 1 1
  spline S565 degree 3 poles (-14.9271, 0.3642) (-14.9451, 0.4274) (-14.9451, 0.5357) (-14.9271, 0.5898) knots 0 0 0 0 1 1 1 1
  spline S566 degree 3 poles (-13.7177, 0.5176) (-13.7448, 0.5898) (-13.7087, 0.671) (-13.6275, 0.6981) knots 0 0 0 0 1 1 1 1
  spline S567 degree 3 poles (-13.6275, 0.6981) (-13.5372, 0.7342) (-13.5101, 0.8245) (-13.5462, 0.9779) knots 0 0 0 0 1 1 1 1
  spline S568 degree 3 poles (-13.5462, 0.9779) (-13.5823, 1.1042) (-13.5643, 1.2035) (-13.5101, 1.2035) knots 0 0 0 0 1 1 1 1
  spline S569 degree 3 poles (-13.5101, 1.2035) (-13.3296, 1.2035) (-13.4199, 1.4562) (-13.6184, 1.5104) knots 0 0 0 0 1 1 1 1
  spline S570 degree 3 poles (-13.6184, 1.5104) (-13.817, 1.5555) (-13.817, 1.5645) (-13.6455, 1.6909) knots 0 0 0 0 1 1 1 1
  spline S571 degree 3 poles (-13.6455, 1.6909) (-13.4831, 1.8082) (-13.456, 1.8082) (-13.3928, 1.6909) knots 0 0 0 0 1 1 1 1
  spline S572 degree 3 poles (-13.3928, 1.6909) (-13.2845, 1.4923) (-13.2935, 1.1042) (-13.4109, 0.7252) knots 0 0 0 0 1 1 1 1
  spline S573 degree 3 poles (-13.4109, 0.7252) (-13.5282, 0.3732) (-13.6365, 0.301) (-13.7177, 0.5176) knots 0 0 0 0 1 1 1 1
  spline S574 degree 3 poles (-18.9703, 0.6169) (-18.519, 0.7793) (-18.4739, 0.7793) (-18.6905, 0.6169) knots 0 0 0 0 1 1 1 1
  spline S575 degree 3 poles (-18.6905, 0.6169) (-18.7898, 0.5447) (-18.9703, 0.4815) (-19.0966, 0.4815) knots 0 0 0 0 1 1 1 1
  spline S576 degree 3 poles (-19.0966, 0.4815) (-19.2952, 0.4905) (-19.2681, 0.5086) (-18.9703, 0.6169) knots 0 0 0 0 1 1 1 1
  spline S577 degree 3 poles (-20.8204, 0.5627) (-20.8204, 0.644) (-20.4504, 0.7703) (-20.3782, 0.7071) knots 0 0 0 0 1 1 1 1
  spline S578 degree 3 poles (-20.3782, 0.7071) (-20.3511, 0.671) (-20.6309, 0.5266) (-20.8023, 0.4905) knots 0 0 0 0 1 1 1 1
  spline S579 degree 3 poles (-20.8023, 0.4905) (-20.8114, 0.4815) (-20.8204, 0.5176) (-20.8204, 0.5627) knots 0 0 0 0 1 1 1 1
  spline S580 degree 3 poles (-14.2682, 0.7071) (-14.3675, 0.7793) (-14.4217, 0.8606) (-14.3946, 0.8876) knots 0 0 0 0 1 1 1 1
  spline S581 degree 3 poles (-14.3946, 0.8876) (-14.3675, 0.9147) (-14.2502, 0.8606) (-14.1329, 0.7613) knots 0 0 0 0 1 1 1 1
  spline S582 degree 3 poles (-14.1329, 0.7613) (-13.8892, 0.5537) (-14.0065, 0.5086) (-14.2682, 0.7071) knots 0 0 0 0 1 1 1 1
  spline S583 degree 3 poles (-15.5859, 0.6079) (-15.5859, 0.6259) (-15.5137, 0.6981) (-15.4325, 0.7613) knots 0 0 0 0 1 1 1 1
  spline S584 degree 3 poles (-15.4325, 0.7613) (-15.2881, 0.8786) (-15.279, 0.8696) (-15.3964, 0.7252) knots 0 0 0 0 1 1 1 1
  spline S585 degree 3 poles (-15.3964, 0.7252) (-15.5137, 0.5808) (-15.5859, 0.5357) (-15.5859, 0.6079) knots 0 0 0 0 1 1 1 1
  spline S586 degree 3 poles (-15.9469, 0.8245) (-15.9469, 0.8696) (-15.8476, 0.9508) (-15.7213, 1.005) knots 0 0 0 0 1 1 1 1
  spline S587 degree 3 poles (-15.7213, 1.005) (-15.4686, 1.1223) (-15.4054, 0.9959) (-15.6581, 0.8515) knots 0 0 0 0 1 1 1 1
  spline S588 degree 3 poles (-15.6581, 0.8515) (-15.8476, 0.7342) (-15.9469, 0.7252) (-15.9469, 0.8245) knots 0 0 0 0 1 1 1 1
  spline S589 degree 3 poles (-13.9704, 1.005) (-13.9072, 1.023) (-13.808, 0.9959) (-13.7628, 0.9508) knots 0 0 0 0 1 1 1 1
  spline S590 degree 3 poles (-13.7628, 0.9508) (-13.6906, 0.8786) (-13.7267, 0.8696) (-13.8802, 0.9057) knots 0 0 0 0 1 1 1 1
  spline S591 degree 3 poles (-13.8802, 0.9057) (-13.9975, 0.9418) (-14.0426, 0.9779) (-13.9704, 1.005) knots 0 0 0 0 1 1 1 1
  spline S592 degree 3 poles (-19.223, 0.9959) (-19.1598, 1.014) (-19.0515, 1.014) (-18.9973, 0.9959) knots 0 0 0 0 1 1 1 1
  spline S593 degree 3 poles (-18.9973, 0.9959) (-18.9342, 0.9689) (-18.9793, 0.9508) (-19.1056, 0.9508) knots 0 0 0 0 1 1 1 1
  spline S594 degree 3 poles (-19.1056, 0.9508) (-19.232, 0.9508) (-19.2771, 0.9689) (-19.223, 0.9959) knots 0 0 0 0 1 1 1 1
  spline S595 degree 3 poles (-19.2591, 1.1674) (-19.232, 1.1945) (-19.1508, 1.2035) (-19.0876, 1.1764) knots 0 0 0 0 1 1 1 1
  spline S596 degree 3 poles (-19.0876, 1.1764) (-19.0154, 1.1494) (-19.0425, 1.1223) (-19.1417, 1.1223) knots 0 0 0 0 1 1 1 1
  spline S597 degree 3 poles (-19.1417, 1.1223) (-19.241, 1.1133) (-19.2952, 1.1403) (-19.2591, 1.1674) knots 0 0 0 0 1 1 1 1
  spline S598 degree 3 poles (-16.0371, 1.3479) (-16.0371, 1.366) (-15.9108, 1.384) (-15.7574, 1.384) knots 0 0 0 0 1 1 1 1
  spline S599 degree 3 poles (-15.7574, 1.384) (-15.613, 1.384) (-15.5047, 1.3479) (-15.5317, 1.3028) knots 0 0 0 0 1 1 1 1
  spline S600 degree 3 poles (-15.5317, 1.3028) (-15.5769, 1.2306) (-16.0371, 1.2757) (-16.0371, 1.3479) knots 0 0 0 0 1 1 1 1
  spline S601 degree 3 poles (-14.0787, 1.3569) (-14.0155, 1.375) (-13.9072, 1.375) (-13.8531, 1.3569) knots 0 0 0 0 1 1 1 1
  spline S602 degree 3 poles (-13.8531, 1.3569) (-13.7899, 1.3299) (-13.835, 1.3118) (-13.9614, 1.3118) knots 0 0 0 0 1 1 1 1
  spline S603 degree 3 poles (-13.9614, 1.3118) (-14.0877, 1.3118) (-14.1329, 1.3299) (-14.0787, 1.3569) knots 0 0 0 0 1 1 1 1
  spline S604 degree 3 poles (-24.8816, 1.375) (-24.8816, 1.4201) (-24.9087, 1.5284) (-24.9448, 1.6187) knots 0 0 0 0 1 1 1 1
  spline S605 degree 3 poles (-24.9448, 1.6187) (-24.9899, 1.745) (-24.9719, 1.7631) (-24.8546, 1.7179) knots 0 0 0 0 1 1 1 1
  spline S606 degree 3 poles (-24.8546, 1.7179) (-24.7192, 1.6638) (-24.7102, 1.6818) (-24.8004, 1.8443) knots 0 0 0 0 1 1 1 1
  spline S607 degree 3 poles (-24.8004, 1.8443) (-24.9538, 2.1421) (-24.8365, 2.1331) (-24.5748, 1.8353) knots 0 0 0 0 1 1 1 1
  spline S608 degree 3 poles (-24.5748, 1.8353) (-24.3311, 1.5465) (-24.3311, 1.2847) (-24.5748, 1.4833) knots 0 0 0 0 1 1 1 1
  spline S609 degree 3 poles (-24.5748, 1.4833) (-24.6831, 1.5735) (-24.6921, 1.5645) (-24.647, 1.4382) knots 0 0 0 0 1 1 1 1
  spline S610 degree 3 poles (-24.647, 1.4382) (-24.6109, 1.3389) (-24.638, 1.2938) (-24.7372, 1.2938) knots 0 0 0 0 1 1 1 1
  spline S611 degree 3 poles (-24.7372, 1.2938) (-24.8185, 1.2938) (-24.8816, 1.3299) (-24.8816, 1.375) knots 0 0 0 0 1 1 1 1
  spline S612 degree 3 poles (27.2197, 2.1331) (27.1926, 2.458) (27.2106, 2.7829) (27.2648, 2.8822) knots 0 0 0 0 1 1 1 1
  spline S613 degree 3 poles (27.2648, 2.8822) (27.3641, 3.0627) (27.3731, 3.0536) (27.6077, 2.4219) knots 0 0 0 0 1 1 1 1
  spline S614 degree 3 poles (27.6077, 2.4219) (27.7251, 2.106) (27.707, 1.7089) (27.5626, 1.5374) knots 0 0 0 0 1 1 1 1
  spline S615 degree 3 poles (27.5626, 1.5374) (27.3641, 1.3028) (27.2738, 1.4652) (27.2197, 2.1331) knots 0 0 0 0 1 1 1 1
  spline S616 degree 3 poles (26.5157, 1.8353) (26.3623, 2.0067) (26.2991, 2.81) (26.4255, 3.0085) knots 0 0 0 0 1 1 1 1
  spline S617 degree 3 poles (26.4255, 3.0085) (26.5608, 3.2251) (26.624, 3.0627) (26.5789, 2.6385) knots 0 0 0 0 1 1 1 1
  spline S618 degree 3 poles (26.5789, 2.6385) (26.5518, 2.3046) (26.5608, 2.1872) (26.6421, 2.2324) knots 0 0 0 0 1 1 1 1
  spline S619 degree 3 poles (26.6421, 2.2324) (26.6962, 2.2685) (26.7413, 2.3768) (26.7413, 2.467) knots 0 0 0 0 1 1 1 1
  spline S620 degree 3 poles (26.7413, 2.467) (26.7413, 2.5573) (26.7774, 2.6656) (26.8316, 2.6926) knots 0 0 0 0 1 1 1 1
  spline S621 degree 3 poles (26.8316, 2.6926) (26.8857, 2.7287) (26.9218, 2.6385) (26.9218, 2.4941) knots 0 0 0 0 1 1 1 1
  spline S622 degree 3 poles (26.9218, 2.4941) (26.9218, 2.3587) (26.9489, 2.088) (26.976, 1.9075) knots 0 0 0 0 1 1 1 1
  spline S623 degree 3 poles (26.976, 1.9075) (27.0301, 1.6096) (27.0211, 1.5826) (26.8496, 1.6277) knots 0 0 0 0 1 1 1 1
  spline S624 degree 3 poles (26.8496, 1.6277) (26.7504, 1.6548) (26.5969, 1.745) (26.5157, 1.8353) knots 0 0 0 0 1 1 1 1
  spline S625 degree 3 poles (-14.1058, 1.6999) (-14.0065, 1.7721) (-13.8802, 1.8353) (-13.835, 1.8353) knots 0 0 0 0 1 1 1 1
  spline S626 degree 3 poles (-13.835, 1.8353) (-13.7809, 1.8353) (-13.817, 1.7721) (-13.9072, 1.6999) knots 0 0 0 0 1 1 1 1
  spline S627 degree 3 poles (-13.9072, 1.6999) (-14.0065, 1.6277) (-14.1329, 1.5645) (-14.178, 1.5645) knots 0 0 0 0 1 1 1 1
  spline S628 degree 3 poles (-14.178, 1.5645) (-14.2321, 1.5645) (-14.196, 1.6277) (-14.1058, 1.6999) knots 0 0 0 0 1 1 1 1
  spline S629 degree 3 poles (-24.4484, 1.8082) (-24.647, 2.0609) (-24.647, 2.4309) (-24.4304, 2.4309) knots 0 0 0 0 1 1 1 1
  spline S630 degree 3 poles (-24.4304, 2.4309) (-24.3401, 2.4309) (-24.277, 2.4129) (-24.304, 2.3858) knots 0 0 0 0 1 1 1 1
  spline S631 degree 3 poles (-24.304, 2.3858) (-24.3221, 2.3677) (-24.2499, 2.2414) (-24.1416, 2.1241) knots 0 0 0 0 1 1 1 1
  spline S632 degree 3 poles (-24.1416, 2.1241) (-23.9791, 1.9436) (-23.9701, 1.9075) (-24.0965, 1.9526) knots 0 0 0 0 1 1 1 1
  spline S633 degree 3 poles (-24.0965, 1.9526) (-24.5658, 2.1331) (-24.5658, 2.1331) (-24.3672, 1.9345) knots 0 0 0 0 1 1 1 1
  spline S634 degree 3 poles (-24.3672, 1.9345) (-24.2499, 1.8262) (-24.1596, 1.7179) (-24.1596, 1.6999) knots 0 0 0 0 1 1 1 1
  spline S635 degree 3 poles (-24.1596, 1.6999) (-24.1596, 1.6006) (-24.3221, 1.6638) (-24.4484, 1.8082) knots 0 0 0 0 1 1 1 1
  spline S636 degree 3 poles (-29.6649, 2.106) (-30.0078, 2.106) (-30.3147, 2.0338) (-30.6486, 1.8804) knots 0 0 0 0 1 1 1 1
  spline S637 degree 3 poles (-30.6486, 1.8804) (-31.1721, 1.6367) (-31.2443, 1.6548) (-31.3345, 2.0338) knots 0 0 0 0 1 1 1 1
  spline S638 degree 3 poles (-31.3345, 2.0338) (-31.3796, 2.2233) (-31.3616, 2.2775) (-31.2082, 2.3316) knots 0 0 0 0 1 1 1 1
  spline S639 degree 3 poles (-31.2082, 2.3316) (-31.0999, 2.3587) (-30.9374, 2.3587) (-30.8381, 2.3316) knots 0 0 0 0 1 1 1 1
  spline S640 degree 3 poles (-30.8381, 2.3316) (-30.7298, 2.2955) (-30.5584, 2.3316) (-30.432, 2.4129) knots 0 0 0 0 1 1 1 1
  spline S641 degree 3 poles (-30.432, 2.4129) (-30.2064, 2.5663) (-29.6829, 2.5934) (-29.1053, 2.5031) knots 0 0 0 0 1 1 1 1
  spline S642 degree 3 poles (-29.1053, 2.5031) (-28.8436, 2.458) (-28.7263, 2.3677) (-28.5819, 2.1331) knots 0 0 0 0 1 1 1 1
  spline S643 degree 3 poles (-28.5819, 2.1331) (-28.3202, 1.6818) (-28.3563, 1.6367) (-28.7895, 1.8804) knots 0 0 0 0 1 1 1 1
  spline S644 degree 3 poles (-28.7895, 1.8804) (-29.0602, 2.0428) (-29.3039, 2.106) (-29.6649, 2.106) knots 0 0 0 0 1 1 1 1
  spline S645 degree 3 poles (-14.3675, 1.9255) (-14.2773, 2.0248) (-14.187, 2.088) (-14.1599, 2.0609) knots 0 0 0 0 1 1 1 1
  spline S646 degree 3 poles (-14.1599, 2.0609) (-14.0968, 2.0067) (-14.3224, 1.745) (-14.4397, 1.745) knots 0 0 0 0 1 1 1 1
  spline S647 degree 3 poles (-14.4397, 1.745) (-14.4848, 1.745) (-14.4578, 1.8262) (-14.3675, 1.9255) knots 0 0 0 0 1 1 1 1
  spline S648 degree 3 poles (-13.808, 2.1692) (-13.7719, 2.2504) (-13.826, 2.3136) (-13.9524, 2.3497) knots 0 0 0 0 1 1 1 1
  spline S649 degree 3 poles (-13.9524, 2.3497) (-14.169, 2.4038) (-14.2141, 2.5573) (-14.0155, 2.5573) knots 0 0 0 0 1 1 1 1
  spline S650 degree 3 poles (-14.0155, 2.5573) (-13.8892, 2.5573) (-13.5101, 2.1511) (-13.5101, 2.0158) knots 0 0 0 0 1 1 1 1
  spline S651 degree 3 poles (-13.5101, 2.0158) (-13.5101, 1.9706) (-13.5914, 1.9616) (-13.6816, 1.9887) knots 0 0 0 0 1 1 1 1
  spline S652 degree 3 poles (-13.6816, 1.9887) (-13.7899, 2.0158) (-13.835, 2.088) (-13.808, 2.1692) knots 0 0 0 0 1 1 1 1
  spline S653 degree 3 poles (-15.5859, 2.5302) (-15.5859, 2.5482) (-15.5498, 2.5573) (-15.4956, 2.5573) knots 0 0 0 0 1 1 1 1
  spline S654 degree 3 poles (-15.4956, 2.5573) (-15.4144, 2.5573) (-15.1346, 2.097) (-15.1346, 1.9616) knots 0 0 0 0 1 1 1 1
  spline S655 degree 3 poles (-15.1346, 1.9616) (-15.1346, 1.9165) (-15.2339, 2.0248) (-15.3603, 2.1963) knots 0 0 0 0 1 1 1 1
  spline S656 degree 3 poles (-15.3603, 2.1963) (-15.4866, 2.3677) (-15.5859, 2.5121) (-15.5859, 2.5302) knots 0 0 0 0 1 1 1 1
  spline S657 degree 3 poles (17.7705, 2.3407) (16.9131, 2.9002) (17.229, 4.4435) (18.2759, 4.8045) knots 0 0 0 0 1 1 1 1
  spline S658 degree 3 poles (18.2759, 4.8045) (18.5106, 4.8857) (18.5286, 4.8767) (18.5286, 4.6601) knots 0 0 0 0 1 1 1 1
  spline S659 degree 3 poles (18.5286, 4.6601) (18.5286, 4.4615) (18.5015, 4.4345) (18.294, 4.4796) knots 0 0 0 0 1 1 1 1
  spline S660 degree 3 poles (18.294, 4.4796) (18.1135, 4.5067) (18.0413, 4.4796) (18.0142, 4.3532) knots 0 0 0 0 1 1 1 1
  spline S661 degree 3 poles (18.0142, 4.3532) (17.9871, 4.254) (17.933, 4.1818) (17.8878, 4.1818) knots 0 0 0 0 1 1 1 1
  spline S662 degree 3 poles (17.8878, 4.1818) (17.8427, 4.1818) (17.8066, 4.0825) (17.8066, 3.9561) knots 0 0 0 0 1 1 1 1
  spline S663 degree 3 poles (17.8066, 3.9561) (17.8066, 3.8117) (17.7525, 3.7305) (17.6712, 3.7305) knots 0 0 0 0 1 1 1 1
  spline S664 degree 3 poles (17.6712, 3.7305) (17.599, 3.7305) (17.5359, 3.6673) (17.5359, 3.5951) knots 0 0 0 0 1 1 1 1
  spline S665 degree 3 poles (17.5359, 3.5951) (17.5359, 3.5139) (17.6171, 3.4598) (17.7344, 3.4598) knots 0 0 0 0 1 1 1 1
  spline S666 degree 3 poles (17.7344, 3.4598) (17.933, 3.4507) (17.933, 3.4507) (17.7705, 3.3244) knots 0 0 0 0 1 1 1 1
  spline S667 degree 3 poles (17.7705, 3.3244) (17.572, 3.18) (17.6442, 2.8731) (17.8517, 2.9544) knots 0 0 0 0 1 1 1 1
  spline S668 degree 3 poles (17.8517, 2.9544) (17.96, 2.9905) (17.9781, 2.9544) (17.933, 2.7829) knots 0 0 0 0 1 1 1 1
  spline S669 degree 3 poles (17.933, 2.7829) (17.8878, 2.6024) (17.9149, 2.5573) (18.0593, 2.5573) knots 0 0 0 0 1 1 1 1
  spline S670 degree 3 poles (18.0593, 2.5573) (18.1586, 2.5573) (18.2669, 2.4941) (18.294, 2.4129) knots 0 0 0 0 1 1 1 1
  spline S671 degree 3 poles (18.294, 2.4129) (18.3481, 2.2775) (18.3662, 2.2775) (18.5196, 2.4129) knots 0 0 0 0 1 1 1 1
  spline S672 degree 3 poles (18.5196, 2.4129) (18.673, 2.5573) (18.6911, 2.5573) (18.7362, 2.3587) knots 0 0 0 0 1 1 1 1
  spline S673 degree 3 poles (18.7362, 2.3587) (18.7723, 2.2504) (18.7452, 2.1331) (18.7001, 2.097) knots 0 0 0 0 1 1 1 1
  spline S674 degree 3 poles (18.7001, 2.097) (18.5557, 2.0158) (18.0683, 2.1421) (17.7705, 2.3407) knots 0 0 0 0 1 1 1 1
  spline S675 degree 3 poles (19.043, 2.2955) (19.0791, 2.4129) (19.1243, 2.449) (19.1784, 2.3948) knots 0 0 0 0 1 1 1 1
  spline S676 degree 3 poles (19.1784, 2.3948) (19.2777, 2.2955) (19.2055, 2.106) (19.0701, 2.106) knots 0 0 0 0 1 1 1 1
  spline S677 degree 3 poles (19.0701, 2.106) (19.034, 2.106) (19.016, 2.1872) (19.043, 2.2955) knots 0 0 0 0 1 1 1 1
  spline S678 degree 3 poles (-25.4683, 2.1692) (-25.369, 2.1963) (-25.2336, 2.2594) (-25.1704, 2.3136) knots 0 0 0 0 1 1 1 1
  spline S679 degree 3 poles (-25.1704, 2.3136) (-25.0351, 2.4219) (-24.9268, 2.3407) (-25.017, 2.2053) knots 0 0 0 0 1 1 1 1
  spline S680 degree 3 poles (-25.017, 2.2053) (-25.0441, 2.1511) (-25.2065, 2.115) (-25.36, 2.115) knots 0 0 0 0 1 1 1 1
  spline S681 degree 3 poles (-25.36, 2.115) (-25.5495, 2.1241) (-25.5856, 2.1421) (-25.4683, 2.1692) knots 0 0 0 0 1 1 1 1
  spline S682 degree 3 poles (-25.9646, 2.1963) (-25.9646, 2.2414) (-25.9285, 2.2865) (-25.8834, 2.2865) knots 0 0 0 0 1 1 1 1
  spline S683 degree 3 poles (-25.8834, 2.2865) (-25.8293, 2.2865) (-25.7661, 2.2414) (-25.739, 2.1963) knots 0 0 0 0 1 1 1 1
  spline S684 degree 3 poles (-25.739, 2.1963) (-25.7119, 2.1421) (-25.748, 2.106) (-25.8202, 2.106) knots 0 0 0 0 1 1 1 1
  spline S685 degree 3 poles (-25.8202, 2.106) (-25.9015, 2.106) (-25.9646, 2.1421) (-25.9646, 2.1963) knots 0 0 0 0 1 1 1 1
  spline S686 degree 3 poles (-26.8942, 2.6114) (-27.0296, 2.7378) (-27.1379, 2.9183) (-27.1379, 2.9995) knots 0 0 0 0 1 1 1 1
  spline S687 degree 3 poles (-27.1379, 2.9995) (-27.1379, 3.2522) (-27.0296, 3.55) (-26.9393, 3.55) knots 0 0 0 0 1 1 1 1
  spline S688 degree 3 poles (-26.9393, 3.55) (-26.8942, 3.55) (-26.8762, 3.4688) (-26.9123, 3.3785) knots 0 0 0 0 1 1 1 1
  spline S689 degree 3 poles (-26.9123, 3.3785) (-26.9484, 3.2522) (-26.9123, 3.189) (-26.7769, 3.1439) knots 0 0 0 0 1 1 1 1
  spline S690 degree 3 poles (-26.7769, 3.1439) (-26.5964, 3.0897) (-26.5874, 3.0807) (-26.7498, 2.9544) knots 0 0 0 0 1 1 1 1
  spline S691 degree 3 poles (-26.7498, 2.9544) (-26.9032, 2.837) (-26.9032, 2.828) (-26.7137, 2.7739) knots 0 0 0 0 1 1 1 1
  spline S692 degree 3 poles (-26.7137, 2.7739) (-26.5964, 2.7468) (-26.5061, 2.6565) (-26.5061, 2.5934) knots 0 0 0 0 1 1 1 1
  spline S693 degree 3 poles (-26.5061, 2.5934) (-26.5061, 2.5212) (-26.443, 2.467) (-26.3708, 2.467) knots 0 0 0 0 1 1 1 1
  spline S694 degree 3 poles (-26.3708, 2.467) (-26.2354, 2.467) (-26.1903, 2.3587) (-26.2895, 2.2594) knots 0 0 0 0 1 1 1 1
  spline S695 degree 3 poles (-26.2895, 2.2594) (-26.3708, 2.1782) (-26.5964, 2.3136) (-26.8942, 2.6114) knots 0 0 0 0 1 1 1 1
  spline S696 degree 3 poles (-26.1451, 2.3497) (-26.1451, 2.3948) (-26.082, 2.5031) (-26.0098, 2.5934) knots 0 0 0 0 1 1 1 1
  spline S697 degree 3 poles (-26.0098, 2.5934) (-25.8744, 2.7739) (-25.8744, 2.7739) (-25.8744, 2.5934) knots 0 0 0 0 1 1 1 1
  spline S698 degree 3 poles (-25.8744, 2.5934) (-25.8744, 2.4851) (-25.9015, 2.3768) (-25.9376, 2.3497) knots 0 0 0 0 1 1 1 1
  spline S699 degree 3 poles (-25.9376, 2.3497) (-26.0188, 2.2685) (-26.1451, 2.2685) (-26.1451, 2.3497) knots 0 0 0 0 1 1 1 1
  spline S700 degree 3 poles (19.4401, 2.7648) (19.4311, 2.8009) (19.5123, 2.7829) (19.6026, 2.7197) knots 0 0 0 0 1 1 1 1
  spline S701 degree 3 poles (19.6026, 2.7197) (19.747, 2.6295) (19.756, 2.5843) (19.6748, 2.4851) knots 0 0 0 0 1 1 1 1
  spline S702 degree 3 poles (19.6748, 2.4851) (19.5936, 2.3768) (19.5665, 2.3858) (19.5123, 2.5302) knots 0 0 0 0 1 1 1 1
  spline S703 degree 3 poles (19.5123, 2.5302) (19.4762, 2.6204) (19.4401, 2.7197) (19.4401, 2.7648) knots 0 0 0 0 1 1 1 1
  spline S704 degree 3 poles (-25.4683, 2.467) (-25.4953, 2.5121) (-25.4863, 2.5573) (-25.4322, 2.5573) knots 0 0 0 0 1 1 1 1
  spline S705 degree 3 poles (-25.4322, 2.5573) (-25.387, 2.5573) (-25.3148, 2.5121) (-25.2878, 2.467) knots 0 0 0 0 1 1 1 1
  spline S706 degree 3 poles (-25.2878, 2.467) (-25.2607, 2.4129) (-25.2697, 2.3768) (-25.3239, 2.3768) knots 0 0 0 0 1 1 1 1
  spline S707 degree 3 poles (-25.3239, 2.3768) (-25.369, 2.3768) (-25.4412, 2.4129) (-25.4683, 2.467) knots 0 0 0 0 1 1 1 1
  spline S708 degree 3 poles (-31.6504, 2.6114) (-31.8309, 2.9363) (-31.6775, 3.0085) (-30.8381, 3.0085) knots 0 0 0 0 1 1 1 1
  spline S709 degree 3 poles (-30.8381, 3.0085) (-30.3688, 3.0085) (-30.2064, 3.0356) (-30.2966, 3.0988) knots 0 0 0 0 1 1 1 1
  spline S710 degree 3 poles (-30.2966, 3.0988) (-30.3688, 3.1439) (-30.6306, 3.189) (-30.8652, 3.189) knots 0 0 0 0 1 1 1 1
  spline S711 degree 3 poles (-30.8652, 3.189) (-31.136, 3.189) (-31.2804, 3.2251) (-31.2443, 3.2793) knots 0 0 0 0 1 1 1 1
  spline S712 degree 3 poles (-31.2443, 3.2793) (-31.1721, 3.3966) (-30.5223, 3.3966) (-29.7551, 3.2702) knots 0 0 0 0 1 1 1 1
  spline S713 degree 3 poles (-29.7551, 3.2702) (-29.2407, 3.18) (-29.1234, 3.1258) (-29.0422, 2.9453) knots 0 0 0 0 1 1 1 1
  spline S714 degree 3 poles (-29.0422, 2.9453) (-28.988, 2.828) (-28.9429, 2.7197) (-28.9429, 2.7017) knots 0 0 0 0 1 1 1 1
  spline S715 degree 3 poles (-28.9429, 2.7017) (-28.9429, 2.6926) (-29.34, 2.6746) (-29.8273, 2.6746) knots 0 0 0 0 1 1 1 1
  spline S716 degree 3 poles (-29.8273, 2.6746) (-30.3598, 2.6656) (-30.8472, 2.6114) (-31.0638, 2.5212) knots 0 0 0 0 1 1 1 1
  spline S717 degree 3 poles (-31.0638, 2.5212) (-31.5421, 2.3497) (-31.515, 2.3407) (-31.6504, 2.6114) knots 0 0 0 0 1 1 1 1
  spline S718 degree 3 poles (-14.6834, 2.7558) (-14.6834, 2.7829) (-14.6022, 2.7919) (-14.5029, 2.7648) knots 0 0 0 0 1 1 1 1
  spline S719 degree 3 poles (-14.5029, 2.7648) (-14.3585, 2.7287) (-14.3404, 2.6926) (-14.4217, 2.5843) knots 0 0 0 0 1 1 1 1
  spline S720 degree 3 poles (-14.4217, 2.5843) (-14.5119, 2.4851) (-14.548, 2.4851) (-14.6022, 2.5753) knots 0 0 0 0 1 1 1 1
  spline S721 degree 3 poles (-14.6022, 2.5753) (-14.6473, 2.6385) (-14.6834, 2.7197) (-14.6834, 2.7558) knots 0 0 0 0 1 1 1 1
  spline S722 degree 3 poles (-15.2971, 2.5753) (-15.4595, 2.7378) (-15.4325, 2.828) (-15.2249, 2.828) knots 0 0 0 0 1 1 1 1
  spline S723 degree 3 poles (-15.2249, 2.828) (-15.1076, 2.828) (-15.0444, 2.7648) (-15.0444, 2.6475) knots 0 0 0 0 1 1 1 1
  spline S724 degree 3 poles (-15.0444, 2.6475) (-15.0444, 2.4399) (-15.1346, 2.4129) (-15.2971, 2.5753) knots 0 0 0 0 1 1 1 1
  spline S725 degree 3 poles (19.1604, 2.81) (19.1604, 2.9453) (19.1784, 2.9453) (19.2506, 2.828) knots 0 0 0 0 1 1 1 1
  spline S726 degree 3 poles (19.2506, 2.828) (19.3679, 2.6475) (19.3679, 2.5302) (19.2506, 2.6024) knots 0 0 0 0 1 1 1 1
  spline S727 degree 3 poles (19.2506, 2.6024) (19.1965, 2.6295) (19.1604, 2.7287) (19.1604, 2.81) knots 0 0 0 0 1 1 1 1
  spline S728 degree 3 poles (18.9167, 2.7558) (18.9438, 2.828) (18.9708, 2.8009) (18.9708, 2.7017) knots 0 0 0 0 1 1 1 1
  spline S729 degree 3 poles (18.9708, 2.7017) (18.9799, 2.6024) (18.9528, 2.5482) (18.9257, 2.5843) knots 0 0 0 0 1 1 1 1
  spline S730 degree 3 poles (18.9257, 2.5843) (18.8986, 2.6114) (18.8896, 2.6926) (18.9167, 2.7558) knots 0 0 0 0 1 1 1 1
  spline S731 degree 3 poles (18.4384, 2.7378) (18.4925, 2.837) (18.5737, 2.9183) (18.6189, 2.9183) knots 0 0 0 0 1 1 1 1
  spline S732 degree 3 poles (18.6189, 2.9183) (18.673, 2.9183) (18.664, 2.837) (18.6008, 2.7378) knots 0 0 0 0 1 1 1 1
  spline S733 degree 3 poles (18.6008, 2.7378) (18.5376, 2.6385) (18.4564, 2.5573) (18.4113, 2.5573) knots 0 0 0 0 1 1 1 1
  spline S734 degree 3 poles (18.4113, 2.5573) (18.3752, 2.5573) (18.3842, 2.6385) (18.4384, 2.7378) knots 0 0 0 0 1 1 1 1
  spline S735 degree 3 poles (-25.4231, 2.8461) (-25.4231, 2.9002) (-25.36, 2.8912) (-25.2878, 2.828) knots 0 0 0 0 1 1 1 1
  spline S736 degree 3 poles (-25.2878, 2.828) (-25.2156, 2.7648) (-25.1524, 2.6746) (-25.1524, 2.6295) knots 0 0 0 0 1 1 1 1
  spline S737 degree 3 poles (-25.1524, 2.6295) (-25.1524, 2.5753) (-25.2156, 2.5843) (-25.2878, 2.6475) knots 0 0 0 0 1 1 1 1
  spline S738 degree 3 poles (-25.2878, 2.6475) (-25.36, 2.7107) (-25.4231, 2.8009) (-25.4231, 2.8461) knots 0 0 0 0 1 1 1 1
  spline S739 degree 3 poles (20.83, 2.828) (20.8029, 2.8731) (20.8119, 2.9183) (20.8661, 2.9183) knots 0 0 0 0 1 1 1 1
  spline S740 degree 3 poles (20.8661, 2.9183) (20.9112, 2.9183) (20.9834, 2.8731) (21.0105, 2.828) knots 0 0 0 0 1 1 1 1
  spline S741 degree 3 poles (21.0105, 2.828) (21.0375, 2.7739) (21.0285, 2.7378) (20.9744, 2.7378) knots 0 0 0 0 1 1 1 1
  spline S742 degree 3 poles (20.9744, 2.7378) (20.9292, 2.7378) (20.857, 2.7739) (20.83, 2.828) knots 0 0 0 0 1 1 1 1
  spline S743 degree 3 poles (26.9038, 3.0266) (26.967, 3.0897) (27.0121, 3.0988) (27.0121, 3.0446) knots 0 0 0 0 1 1 1 1
  spline S744 degree 3 poles (27.0121, 3.0446) (27.0121, 2.9183) (26.9038, 2.81) (26.8406, 2.8731) knots 0 0 0 0 1 1 1 1
  spline S745 degree 3 poles (26.8406, 2.8731) (26.8226, 2.9002) (26.8496, 2.9724) (26.9038, 3.0266) knots 0 0 0 0 1 1 1 1
  spline S746 degree 3 poles (18.2579, 2.9634) (18.321, 3.0356) (18.4113, 3.0988) (18.4564, 3.0988) knots 0 0 0 0 1 1 1 1
  spline S747 degree 3 poles (18.4564, 3.0988) (18.5106, 3.0988) (18.5015, 3.0356) (18.4384, 2.9634) knots 0 0 0 0 1 1 1 1
  spline S748 degree 3 poles (18.4384, 2.9634) (18.3752, 2.8912) (18.2849, 2.828) (18.2398, 2.828) knots 0 0 0 0 1 1 1 1
  spline S749 degree 3 poles (18.2398, 2.828) (18.1857, 2.828) (18.1947, 2.8912) (18.2579, 2.9634) knots 0 0 0 0 1 1 1 1
  spline S750 degree 3 poles (22.3191, 3.4778) (22.3191, 4.0825) (22.3642, 4.2088) (22.6079, 4.2991) knots 0 0 0 0 1 1 1 1
  spline S751 degree 3 poles (22.6079, 4.2991) (22.7162, 4.3352) (22.7703, 4.3081) (22.7703, 4.2269) knots 0 0 0 0 1 1 1 1
  spline S752 degree 3 poles (22.7703, 4.2269) (22.7703, 3.9832) (22.9238, 4.0915) (22.9869, 4.3713) knots 0 0 0 0 1 1 1 1
  spline S753 degree 3 poles (22.9869, 4.3713) (23.0411, 4.642) (23.0591, 4.6511) (23.3299, 4.5879) knots 0 0 0 0 1 1 1 1
  spline S754 degree 3 poles (23.3299, 4.5879) (23.4923, 4.5518) (23.7089, 4.5247) (23.8082, 4.5247) knots 0 0 0 0 1 1 1 1
  spline S755 degree 3 poles (23.8082, 4.5247) (23.8985, 4.5337) (24.0338, 4.4886) (24.106, 4.4345) knots 0 0 0 0 1 1 1 1
  spline S756 degree 3 poles (24.106, 4.4345) (24.2053, 4.3532) (24.2504, 4.3623) (24.3136, 4.4796) knots 0 0 0 0 1 1 1 1
  spline S757 degree 3 poles (24.3136, 4.4796) (24.3948, 4.615) (24.5663, 4.633) (25.6583, 4.633) knots 0 0 0 0 1 1 1 1
  spline S758 degree 3 poles (25.6583, 4.633) (26.985, 4.633) (27.1926, 4.5969) (27.1926, 4.3893) knots 0 0 0 0 1 1 1 1
  spline S759 degree 3 poles (27.1926, 4.3893) (27.1926, 4.3171) (27.1475, 4.2901) (27.1023, 4.3171) knots 0 0 0 0 1 1 1 1
  spline S760 degree 3 poles (27.1023, 4.3171) (26.976, 4.3984) (26.4706, 4.281) (26.4706, 4.1727) knots 0 0 0 0 1 1 1 1
  spline S761 degree 3 poles (26.4706, 4.1727) (26.4706, 4.1276) (26.6691, 4.0915) (26.9218, 4.0915) knots 0 0 0 0 1 1 1 1
  spline S762 degree 3 poles (26.9218, 4.0915) (27.346, 4.0915) (27.3731, 4.0735) (27.3731, 3.8659) knots 0 0 0 0 1 1 1 1